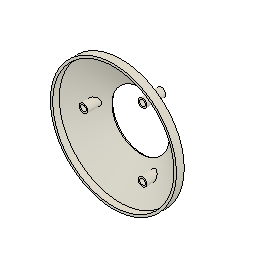
StevensonScreen (Autodesk Fusion 360 archive; units mm, degrees)
design "Shield"
Autodesk Fusion 360 part; units mm, degrees
sketch "Skizze1" plane through (0, 0, 0) normal (0, 1, 0) x (1, 0, 0)
  line L0 (-39.183, 0) -> (-40, 1.258) construction
  line L1 (-40, 1.258) -> (-19.0332, 14.874)
  line L2 (-19.0332, 14.874) -> (-16.31, 10.6806)
  line L3 (-16.31, 10.6806) -> (-17.568, 9.8637)
  line L4 (-17.568, 9.8637) -> (-19.4743, 12.799)
  line L5 (-19.4743, 12.799) -> (-39.183, 0)
  line L6 (0, -20) -> (0, -2.5)
  line L7 (2.5, 0) -> (20, 0)
  line L8 (-40, 1.258) -> (-40, -3.742)
  line L9 (-40, -3.742) -> (-38.5, -3.742)
  line L10 (-38.5, -3.742) -> (-38.5, 0.4436)
  line L11 (-19.4743, 12.799) -> (-18.2163, 13.616)
  dimension "d1" = 1.5
  dimension "d2" = 25
  dimension "d3" = 5
  dimension "d4" = 80
  dimension "d5" = 33
  dimension "d19" = 5
  constraint perpendicular L2 L3
  constraint parallel L1 L5
  constraint parallel L2 L4
  constraint perpendicular L0 L5
  constraint perpendicular L4 L5
  constraint equal L0 L3
  constraint horizontal origin L0.start
  constraint vertical L8
  constraint perpendicular L8 L9
  constraint coincident L5 L10.end
  constraint perpendicular L9 L10
  constraint equal L0 L9
  constraint coincident L2 L11.end
  constraint perpendicular L2 L11
  measures "d1" distance of L0.start L0.end
  measures "d2" distance of L0.end L1.end
  measures "d3" distance of L1.end L2.end
  measures "d5" angle of L5 L7
  measures "d19" distance of L0.end L8.end
revolve "Drehen1" add sketch "Skizze1" angle 360 about axis through (0, 0, 20) along (0, 0, -1) contours L1 L2 L5 L8 L9 L10 L11
ref_plane "Arbeitsebene1" through (0, 0, -8.258) normal (0, 0, 1) x (1, 0, 0)
sketch "Skizze2" plane through (0, 0, -8.258) normal (0, 0, 1) x (1, 0, 0)
  circle A0 centre (-25, 0) radius 2.75
  dimension "d8" = 5.5
  dimension "d9" = 25
  constraint horizontal origin A0.centre
  measures "d8" diameter of A0
  measures "d9" distance of origin A0.centre
extrude "Extrusion1" add sketch "Skizze2" along normal mid plane 12
sketch "Skizze3" plane through (0, 0, -14.258) normal (0, 0, -1) x (-1, 0, 0)
  circle A0 centre (25, 0) radius 2.75
  point P0 (25, 0)
  constraint coincident P0 A0.centre
hole "Bohrung1" at (-25, 0, -14.258) direction (0, 0, 1) diameter 3.6 end through all
fillet "Abrundung1" radius 1 1 edges at (-25.256, -2.7374, -10.7369)
pattern_circular "C-Anordnung1" count 3 over 360 about axis through (0, 0, 1.75) along (0, 0, 1) of "Extrusion1", "Bohrung1", "Abrundung1"

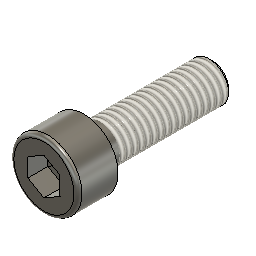
design "Innensechskantschraube ISO 4762 - M5 x 16 Stahl 4.6 Einfach"
description: Innensechskantschraube ISO 4762 - M5 x 16
part number: ISO 4762 - M5 x 16 Stahl 4.6 Einfach
Autodesk Fusion 360 part; units mm, degrees
sketch "Sketch1" plane through (0, 0, 0) normal (0, 1, 0) x (1, 0, 0)
  line L0 (-2.5, 0) -> (-2.5, 16)
  line L1 (-2.5, 16) -> (0, 16)
  line L2 (0, 16) -> (0, -5)
  line L3 (-2.5, 0) -> (-4.25, 0)
  line L4 (-4.25, 0) -> (-4.25, -5)
  line L5 (-4.25, -5) -> (0, -5)
  dimension "d9" = 5
  dimension "d106" = 5
  dimension "d107" = 16
  dimension "d116" = 8.5
  constraint perpendicular L0 L1
  constraint collinear origin L1.end L2.end
  constraint perpendicular L0 L3
  constraint coincident origin L3
  constraint vertical L2
  constraint coincident L2 L5.end
  constraint perpendicular L2 L5
  measures "d106" distance of L3 L5
  measures "d107" distance of origin L1
revolve "Revolve1" add sketch "Sketch1" angle 360 about axis through (0, 0, -16) along (0, 0, 1)
ref_plane "WorkPlane1" through (0, 0, 5) normal (0, 0, 1) x (1, 0, 0)
sketch "Sketch6" plane through (0, 0, 5) normal (0, 0, 1) x (1, 0, 0)
  line L0 (-2, 1.1547) -> (-2, -1.1547)
  line L1 (-2, -1.1547) -> (0, -2.3094)
  line L2 (0, -2.3094) -> (2, -1.1547)
  line L3 (2, -1.1547) -> (2, 1.1547)
  line L4 (2, 1.1547) -> (0, 2.3094)
  line L5 (0, 2.3094) -> (-2, 1.1547)
  dimension "d117" = 4
  constraint vertical L0
  measures "d117" distance of L0 L3
extrude "Extrude1" cut sketch "Sketch6" against normal blind 2.5
extrude "Extrude2" cut 1 faces at (0.6667, -0.3849, 2.5) along direction (0, 0, -1) blind 2.5 draft -85
fillet "Fillet4" radius 0.5 1 edges at (-3.9624, 1.5369, 5)
thread "Thread3" "ISO Metric profile 5.0 M5x0.8 M5x0.8 6g" major diameter 4.901 minor diameter 3.9895 pitch 0.8 angle 60 resizes the face on face at (-2.4876, 0.2489, -10.6667) from (0, 0, -2) to (0, 0, -16)
sketch "Sketch7" plane through (0, 0, 0) normal (0, 1, 0) x (1, 0, 0)
  line L0 (-2.55, 16) -> (-2.55, 15.5)
  line L1 (-2.55, 15.5) -> (-2.05, 16)
  line L2 (0, 16) -> (0, -5)
  line L3 (-2.55, 16) -> (0, 16)
  dimension "d101" = 45
  dimension "d112" = 0.5
  dimension "d113" = 2.55
  constraint coincident L2.start L3.end
  constraint perpendicular L2 L3
  constraint coincident L1.end L3
  constraint perpendicular L0 L3
  measures "d101" angle of L0 L1
  measures "d112" distance of L0.end L3
  measures "d113" distance of L0 L2.start
revolve "Revolve3" cut sketch "Sketch7" angle 360 about axis through (0, 0, 1.75) along (0, 0, 1)
equation "d9 = adsk_nomdia"
equation "adsk_nomlen = 16,00 mm"
equation "adsk_headh = 5,00 mm"
equation "adsk_headdia = 8,50 mm"
equation "adsk_nomdia = 5,00 mm"
equation "adsk_philwidth = 4,00 mm"
equation "d31 = -adsk_phildepth"
equation "adsk_phildepth = 2,50 mm"
equation "d71 = adsk_headh"
equation "d76 = -adsk_phildepth"
equation "adsk_thrlen = 14,00 mm"
equation "d86 = adsk_nomdia * 0,1"
equation "adsk_startang = 45,00 deg"
equation "d101 = adsk_startang"
equation "adsk_pitch1 = 0,80 mm"
equation "adsk_startlen = 0,50 mm"
equation "d106 = adsk_headh"
equation "d107 = adsk_nomlen"
equation "d112 = adsk_startlen"
equation "d113 = adsk_nomdia * 0,51"
equation "d115 = min(adsk_thrlen; adsk_nomlen - 0,001 mm)"
equation "d116 = adsk_headdia"
equation "d117 = adsk_philwidth"

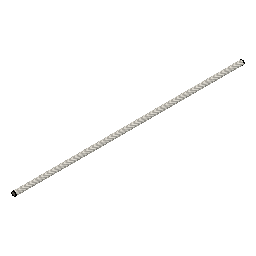
design "Gewindestange"
Autodesk Fusion 360 part; units mm, degrees
sketch "Skizze1" plane through (0, 0, 0) normal (0, 0, 1) x (1, 0, 0)
  circle A0 centre (0, 0) radius 1.5
  dimension "d1" = 3
  constraint coincident A0.centre origin
  measures "d1" diameter of A0
extrude "Extrusion1" add sketch "Skizze1" along normal blind 150
thread "Gewinde1" "ISO Metric profile 3.0 M3x0.5 M3x0.5 6g" major diameter 2.927 minor diameter 2.3555 pitch 0.5 angle 60 resizes the face on face at (-0.989, 1.1278, 100)
chamfer "Fase1" distance 0.25 angle 45 2 edges at (-1.3645, -0.5292, 150) (-1.3645, -0.5292, 0)

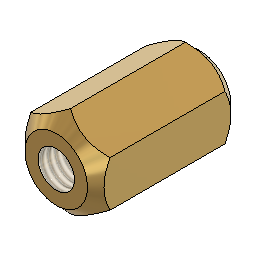
design "Abstandsbolzen"
Autodesk Fusion 360 part; units mm, degrees
sketch "Skizze1" plane through (0, 0, 0) normal (0, 0, 1) x (1, 0, 0)
  line L0 (2.75, 1.5877) -> (0, 3.1754)
  line L1 (0, 3.1754) -> (-2.75, 1.5877)
  line L2 (-2.75, 1.5877) -> (-2.75, -1.5877)
  line L3 (-2.75, -1.5877) -> (0, -3.1754)
  line L4 (0, -3.1754) -> (2.75, -1.5877)
  line L5 (2.75, -1.5877) -> (2.75, 1.5877)
  dimension "d1" = 5.5
  constraint vertical L5
  measures "d1" distance of L2 L5
extrude "Extrusion1" add sketch "Skizze1" along normal blind 10
sketch "Skizze2" plane through (0, 0, 0) normal (1, 0, 0) x (0, 0, -1)
  line L0 (-10, 1.5877) -> (-10, 3.1754)
  line L1 (0, 1.5877) -> (0, 3.1754)
  line L2 (0, 3.1754) -> (-10, 3.1754)
  line L3 (2, 0.1754) -> (-1.5, 3.6754)
  line L4 (-1.5, 3.6754) -> (2, 3.6754)
  line L5 (2, 3.6754) -> (2, 0.1754)
  line L6 (-8.5, 3.6754) -> (-12, 3.6754)
  line L7 (-12, 3.6754) -> (-12, 0.1754)
  line L8 (-12, 0.1754) -> (-8.5, 3.6754)
  dimension "d4" = 45
  dimension "d5" = 45
  dimension "d6" = 2
  dimension "d7" = 2
  dimension "d8" = 3.5
  dimension "d9" = 0.5
  constraint perpendicular L1 L4
  constraint perpendicular L4 L5
  constraint parallel L4 L6
  constraint perpendicular L6 L7
  constraint equal L4 L6
  constraint collinear L4 L6
  measures "d4" angle of L3 L4
  measures "d5" angle of L7 L8
  measures "d6" distance of L0 L7
  measures "d7" horizontal distance of L1.end L4.end
  measures "d8" distance of L6.start L6.end
  measures "d9" distance of L0.end L6
revolve "Drehen1" cut sketch "Skizze2" angle 360 about axis through (0, 0, 1.75) along (0, 0, 1)
hole "Bohrung1" at (0, 0, 10) direction (0, 0, -1) diameter 2.529 end through all
thread "Gewinde1" "ISO Metric profile 3.0 M3x0.5 M3x0.5 6H" thread offset 0 thread depth 7.4
